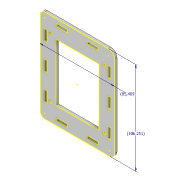
# Autodesk Inventor part: tapa1
Saved by Autodesk Inventor 2019 (Build 230136000, 136)
## iProperties
Created: 2018-09-17
Part Number: tapa1
Material: Genérico
Document SubType Name: Modeling
Designer: lmacia
Density: 1 g/cm^3
Appearance: Valor por defecto
Author: lmacia
Autodesk Inventor part; units mm, degrees
ref_plane "YZ Plane" through (0, 0, 0) normal (1, 0, 0) x (0, 1, 0)
ref_plane "XZ Plane" through (0, 0, 0) normal (0, 1, 0) x (-1, 0, 0)
ref_plane "XY Plane" through (0, 0, 0) normal (0, 0, 1) x (1, 0, 0)
sketch "Boceto1" plane through (0, 0, 0) normal (0, 0, 1) x (-1, 0, 0)
  line L0 (35.0245, 23.8411) -> (34.9228, 23.8411)
  line L1 (34.9228, 23.8411) -> (34.9228, 36.0412)
  line L2 (34.9228, 36.0412) -> (35.0245, 36.0412)
  line L3 (34.9228, 36.0412) -> (37.9729, 36.0412)
  line L4 (38.0745, 36.0412) -> (38.1762, 36.0412)
  line L5 (38.1762, 23.8411) -> (38.0745, 23.8411)
  line L6 (37.9729, 23.8411) -> (34.9228, 23.8411)
  line L7 (34.9937, -6.4559) -> (34.892, -6.4559)
  line L8 (34.892, -6.4559) -> (34.892, 5.7442)
  line L9 (34.892, 5.7442) -> (34.9937, 5.7442)
  line L10 (34.892, 5.7442) -> (38.1762, 5.7442)
  line L11 (38.1762, -6.4559) -> (38.0745, -6.4559)
  line L12 (38.0745, -6.4559) -> (34.9937, -6.4559)
  line L13 (32.3812, 32.3812) -> (32.3327, 32.0128)
  line L14 (32.3327, 32.0128) -> (32.1905, 31.6695)
  line L15 (32.2, 31.6622) -> (31.9738, 31.3674)
  line L16 (31.9643, 31.3747) -> (31.6695, 31.1485)
  line L17 (31.6695, 31.1485) -> (31.3262, 31.0063)
  line L18 (31.3262, 31.0063) -> (30.9578, 30.9578)
  line L19 (30.9578, 30.9578) -> (30.5894, 31.0063)
  line L20 (30.5894, 31.0063) -> (30.2461, 31.1485)
  line L21 (30.2461, 31.1485) -> (29.9513, 31.3747)
  line L22 (29.9418, 31.3674) -> (29.7156, 31.6622)
  line L23 (29.7252, 31.6695) -> (29.583, 32.0128)
  line L24 (29.583, 32.0128) -> (29.5345, 32.3812)
  line L25 (29.5345, 32.3812) -> (29.583, 32.7495)
  line L26 (29.583, 32.7495) -> (29.7252, 33.0928)
  line L27 (29.7252, 33.0928) -> (29.9513, 33.3876)
  line L28 (29.9513, 33.3876) -> (30.2461, 33.6138)
  line L29 (30.2461, 33.6138) -> (30.5894, 33.756)
  line L30 (30.5894, 33.756) -> (30.9578, 33.8045)
  line L31 (30.9594, 33.8164) -> (31.3278, 33.7679)
  line L32 (31.3262, 33.756) -> (31.6695, 33.6138)
  line L33 (31.6695, 33.6138) -> (31.9643, 33.3876)
  line L34 (31.9643, 33.3876) -> (32.1905, 33.0928)
  line L35 (32.1905, 33.0928) -> (32.3327, 32.7495)
  line L36 (32.3327, 32.7495) -> (32.3812, 32.3812)
  line L37 (24.7052, 32.9403) -> (24.7052, -32.9403)
  line L38 (24.7052, -32.9403) -> (-24.7052, -32.9403)
  line L39 (-24.7052, -32.9403) -> (-24.7052, 32.9403)
  line L40 (-24.7052, 32.9403) -> (24.7052, 32.9403)
  line L41 (-35.0245, 36.0412) -> (-34.9228, 36.0412)
  line L42 (-34.9228, 36.0412) -> (-34.9228, 23.8411)
  line L43 (-34.9228, 23.8411) -> (-35.0245, 23.8411)
  line L44 (-35.0245, 23.8411) -> (-38.0745, 23.8411)
  line L45 (-38.0745, 23.8411) -> (-38.1762, 23.8411)
  line L46 (-38.1762, 23.8411) -> (-38.1762, 36.0412)
  line L47 (-38.1762, 36.0412) -> (-38.0745, 36.0412)
  line L48 (-38.0745, 36.0412) -> (-35.0245, 36.0412)
  line L49 (-35.0245, -36.7529) -> (-38.0745, -36.7529)
  line L50 (-38.0745, -36.7529) -> (-38.1762, -36.7529)
  line L51 (-38.1762, -36.7529) -> (-38.1762, -24.5527)
  line L52 (-38.1762, -24.5527) -> (-38.0745, -24.5527)
  line L53 (-38.0745, -24.5527) -> (-35.0245, -24.5527)
  line L54 (-35.0245, -24.5527) -> (-34.9228, -24.5527)
  line L55 (-34.9228, -24.5527) -> (-34.9228, -36.7529)
  line L56 (-34.9228, -36.7529) -> (-35.0245, -36.7529)
  line L57 (-30.5894, 31.0063) -> (-30.9578, 30.9578)
  line L58 (-30.9578, 30.9578) -> (-31.3262, 31.0063)
  line L59 (-31.3262, 31.0063) -> (-31.6695, 31.1485)
  line L60 (-31.6695, 31.1485) -> (-31.9643, 31.3747)
  line L61 (-31.9643, 31.3747) -> (-32.1905, 31.6695)
  line L62 (-32.2016, 31.6649) -> (-32.3438, 32.0082)
  line L63 (-32.3327, 32.0128) -> (-32.3812, 32.3812)
  line L64 (-32.3812, 32.3812) -> (-32.3327, 32.7495)
  line L65 (-32.3327, 32.7495) -> (-32.1905, 33.0928)
  line L66 (-32.1905, 33.0928) -> (-31.9643, 33.3876)
  line L67 (-31.9643, 33.3876) -> (-31.6695, 33.6138)
  line L68 (-31.6695, 33.6138) -> (-31.3262, 33.756)
  line L69 (-31.3262, 33.756) -> (-30.9578, 33.8045)
  line L70 (-30.9562, 33.8164) -> (-30.5878, 33.7679)
  line L71 (-30.5894, 33.756) -> (-30.2461, 33.6138)
  line L72 (-30.2461, 33.6138) -> (-29.9513, 33.3876)
  line L73 (-29.9513, 33.3876) -> (-29.7252, 33.0928)
  line L74 (-29.7252, 33.0928) -> (-29.583, 32.7495)
  line L75 (-29.583, 32.7495) -> (-29.5345, 32.3812)
  line L76 (-29.5345, 32.3812) -> (-29.583, 32.0128)
  line L77 (-29.583, 32.0128) -> (-29.7252, 31.6695)
  line L78 (-29.7252, 31.6695) -> (-29.9513, 31.3747)
  line L79 (-29.9513, 31.3747) -> (-30.2461, 31.1485)
  line L80 (-30.2415, 31.1374) -> (-30.5848, 30.9952)
  line L81 (-38.1762, -6.4559) -> (-38.1762, 5.7442)
  line L82 (-38.1762, 5.7442) -> (-38.0745, 5.7442)
  line L83 (-38.0745, 5.7442) -> (-35.0245, 5.7442)
  line L84 (-35.0245, 5.7442) -> (-34.9228, 5.7442)
  line L85 (-34.9228, 5.7442) -> (-34.9228, -6.4559)
  line L86 (-34.9228, -6.4559) -> (-35.0245, -6.4559)
  line L87 (-35.0245, -6.4559) -> (-38.0745, -6.4559)
  line L88 (-38.0745, -6.4559) -> (-38.1762, -6.4559)
  line L89 (-30.5894, -36.6027) -> (-30.9578, -36.6512)
  line L90 (-30.9578, -36.6512) -> (-31.3262, -36.6027)
  line L91 (-31.3262, -36.6027) -> (-31.6695, -36.4605)
  line L92 (-31.6695, -36.4605) -> (-31.9643, -36.2343)
  line L93 (-31.9643, -36.2343) -> (-32.1905, -35.9395)
  line L94 (-32.2016, -35.9441) -> (-32.3438, -35.6008)
  line L95 (-32.3327, -35.5962) -> (-32.3812, -35.2278)
  line L96 (-32.3812, -35.2278) -> (-32.3327, -34.8595)
  line L97 (-32.3327, -34.8595) -> (-32.1905, -34.5162)
  line L98 (-32.1905, -34.5162) -> (-31.9643, -34.2214)
  line L99 (-31.9643, -34.2214) -> (-31.6695, -33.9952)
  line L100 (-31.6695, -33.9952) -> (-31.3262, -33.853)
  line L101 (-31.3262, -33.853) -> (-30.9578, -33.8045)
  line L102 (-30.9562, -33.7926) -> (-30.5878, -33.8411)
  line L103 (-30.5894, -33.853) -> (-30.2461, -33.9952)
  line L104 (-30.2461, -33.9952) -> (-29.9513, -34.2214)
  line L105 (-29.9513, -34.2214) -> (-29.7252, -34.5162)
  line L106 (-29.7252, -34.5162) -> (-29.583, -34.8595)
  line L107 (-29.583, -34.8595) -> (-29.5345, -35.2278)
  line L108 (-29.5345, -35.2278) -> (-29.583, -35.5962)
  line L109 (-29.583, -35.5962) -> (-29.7252, -35.9395)
  line L110 (-29.7252, -35.9395) -> (-29.9513, -36.2343)
  line L111 (-29.944, -36.2439) -> (-30.2388, -36.4701)
  line L112 (-30.2461, -36.4605) -> (-30.5894, -36.6027)
  line L113 (11.4122, -48.8513) -> (11.4122, -45.8013)
  line L114 (11.4122, -45.8013) -> (11.4122, -45.6996)
  line L115 (11.4122, -45.6996) -> (23.6123, -45.6996)
  line L116 (23.6123, -45.6996) -> (23.6123, -45.8013)
  line L117 (23.6123, -45.8013) -> (23.6123, -48.8513)
  line L118 (23.6123, -48.8513) -> (23.6123, -48.953)
  line L119 (23.6123, -48.953) -> (11.4122, -48.953)
  line L120 (11.4122, -48.953) -> (11.4122, -48.8513)
  line L121 (11.4122, 44.9879) -> (11.4122, 45.0896)
  line L122 (11.4122, 44.9879) -> (11.4122, 48.1396)
  line L123 (11.4122, 48.1396) -> (11.4122, 48.2413)
  line L124 (23.6123, 48.2413) -> (23.6123, 48.1396)
  line L125 (23.6123, 44.9879) -> (11.4122, 44.9879)
  line L126 (-23.6123, 44.9879) -> (-23.6123, 45.0896)
  line L127 (-23.6123, 45.0896) -> (-23.6123, 48.1396)
  line L128 (-23.6123, 48.1396) -> (-23.6123, 48.2413)
  line L129 (-23.6123, 48.2413) -> (-11.4122, 48.2413)
  line L130 (-11.4122, 48.2413) -> (-11.4122, 48.1396)
  line L131 (-11.4122, 48.1396) -> (-11.4122, 45.0896)
  line L132 (-11.4122, 45.0896) -> (-11.4122, 44.9879)
  line L133 (-11.4122, 44.9879) -> (-23.6123, 44.9879)
  line L134 (-11.4122, -45.6996) -> (-11.4122, -45.8013)
  line L135 (-11.4122, -45.8013) -> (-11.4122, -48.8513)
  line L136 (-11.4122, -48.8513) -> (-11.4122, -48.953)
  line L137 (-11.4122, -48.953) -> (-23.6123, -48.953)
  line L138 (-23.6123, -48.953) -> (-23.6123, -48.8513)
  line L139 (-23.6123, -48.8513) -> (-23.6123, -45.8013)
  line L140 (-23.6123, -45.8013) -> (-23.6123, -45.6996)
  line L141 (-23.6123, -45.6996) -> (-11.4122, -45.6996)
  line L142 (32.3327, -34.8595) -> (32.3812, -35.2278)
  line L143 (32.3812, -35.2278) -> (32.3327, -35.5962)
  line L144 (32.3327, -35.5962) -> (32.1905, -35.9395)
  line L145 (32.1905, -35.9395) -> (31.9643, -36.2343)
  line L146 (31.9716, -36.2439) -> (31.6768, -36.4701)
  line L147 (31.6695, -36.4605) -> (31.3262, -36.6027)
  line L148 (31.3262, -36.6027) -> (30.9578, -36.6512)
  line L149 (30.9578, -36.6512) -> (30.5894, -36.6027)
  line L150 (30.5894, -36.6027) -> (30.2461, -36.4605)
  line L151 (30.2461, -36.4605) -> (29.9513, -36.2343)
  line L152 (29.9513, -36.2343) -> (29.7252, -35.9395)
  line L153 (29.7252, -35.9395) -> (29.583, -35.5962)
  line L154 (29.583, -35.5962) -> (29.5345, -35.2278)
  line L155 (29.5345, -35.2278) -> (29.583, -34.8595)
  line L156 (29.583, -34.8595) -> (29.7252, -34.5162)
  line L157 (29.7252, -34.5162) -> (29.9513, -34.2214)
  line L158 (29.944, -34.2118) -> (30.2388, -33.9856)
  line L159 (30.2461, -33.9952) -> (30.5894, -33.853)
  line L160 (30.5894, -33.853) -> (30.9578, -33.8045)
  line L161 (30.9578, -33.8045) -> (31.3262, -33.853)
  line L162 (31.3262, -33.853) -> (31.6695, -33.9952)
  line L163 (31.6768, -33.9856) -> (31.9716, -34.2118)
  line L164 (31.9643, -34.2214) -> (32.1905, -34.5162)
  line L165 (32.1905, -34.5162) -> (32.3327, -34.8595)
  line L166 (34.9228, -36.7529) -> (34.9228, -24.5527)
  line L167 (34.9228, -24.5527) -> (35.0245, -24.5527)
  line L168 (35.0245, -24.5527) -> (38.0745, -24.5527)
  line L169 (38.0745, -24.5527) -> (38.1762, -24.5527)
  line L170 (38.1762, -24.5527) -> (38.1762, -36.7529)
  line L171 (38.1762, -36.7529) -> (38.0745, -36.7529)
  line L172 (38.0745, -36.7529) -> (35.0245, -36.7529)
  line L173 (35.0245, -36.7529) -> (34.9228, -36.7529)
  line L174 (23.6123, -48.953) -> (11.4122, -48.953)
  line L175 (11.4122, -48.953) -> (11.4122, -45.6996)
  line L176 (11.4122, -45.6996) -> (23.6123, -45.6996)
  line L177 (23.6123, -45.6996) -> (23.6123, -48.953)
  line L178 (-11.4122, -48.953) -> (-23.6123, -48.953)
  line L179 (-23.6123, -48.953) -> (-23.6123, -45.6996)
  line L180 (-23.6123, -45.6996) -> (-11.4122, -45.6996)
  line L181 (-11.4122, -45.6996) -> (-11.4122, -48.953)
  line L182 (-34.9228, -36.7529) -> (-38.1762, -36.7529)
  line L183 (-38.1762, -36.7529) -> (-38.1762, -24.5527)
  line L184 (-38.1762, -24.5527) -> (-34.9228, -24.5527)
  line L185 (-34.9228, -24.5527) -> (-34.9228, -36.7529)
  line L186 (-34.9228, -6.4559) -> (-38.1762, -6.4559)
  line L187 (-38.1762, -6.4559) -> (-38.1762, 5.7442)
  line L188 (-38.1762, 5.7442) -> (-34.9228, 5.7442)
  line L189 (-34.9228, 5.7442) -> (-34.9228, -6.4559)
  line L190 (-34.9228, 23.8411) -> (-38.1762, 23.8411)
  line L191 (-38.1762, 23.8411) -> (-38.1762, 36.0412)
  line L192 (-38.1762, 36.0412) -> (-34.9228, 36.0412)
  line L193 (-34.9228, 36.0412) -> (-34.9228, 23.8411)
  line L194 (-23.6123, 44.9879) -> (-11.4122, 44.9879)
  line L195 (-11.4122, 44.9879) -> (-11.4122, 48.2413)
  line L196 (-11.4122, 48.2413) -> (-23.6123, 48.2413)
  line L197 (-23.6123, 48.2413) -> (-23.6123, 44.9879)
  line L198 (11.4122, 44.9879) -> (23.6123, 44.9879)
  line L199 (23.6123, 44.9879) -> (23.6123, 48.2413)
  line L200 (23.6123, 48.2413) -> (11.4122, 48.2413)
  line L201 (11.4122, 48.2413) -> (11.4122, 44.9879)
  line L202 (34.9228, 36.0412) -> (38.1762, 36.0412)
  line L203 (38.1762, 36.0412) -> (38.1762, 23.8411)
  line L204 (38.1762, 23.8411) -> (34.9228, 23.8411)
  line L205 (34.9228, 23.8411) -> (34.9228, 36.0412)
  line L206 (34.892, 5.7442) -> (38.1455, 5.7442)
  line L207 (38.1455, 5.7442) -> (38.1455, -6.4559)
  line L208 (38.1455, -6.4559) -> (34.892, -6.4559)
  line L209 (34.892, -6.4559) -> (34.892, 5.7442)
  line L210 (38.1762, -36.7529) -> (34.9228, -36.7529)
  line L211 (34.9228, -36.7529) -> (34.9228, -24.5527)
  line L212 (34.9228, -24.5527) -> (38.1762, -24.5527)
  line L213 (38.1762, -24.5527) -> (38.1762, -36.7529)
  circle A0 centre (30.9578, 32.3812) radius 1.4232
  circle A1 centre (30.9578, -35.2278) radius 1.4232
  circle A2 centre (-30.9578, -35.2278) radius 1.4232
  circle A3 centre (-30.9578, 32.3812) radius 1.4232
  line L214 (37.2318, -53.5669) -> (-35.5862, -53.5669)
  arc A4 (-42.6187, -46.5344) -> (-35.5862, -53.5669) centre (-35.5862, -46.5344) ccw
  line L215 (-42.6187, -46.5344) -> (-42.6187, 47.1583)
  arc A5 (-37.0932, 52.6838) -> (-42.6187, 47.1583) centre (-37.0932, 47.1583) ccw
  line L216 (-37.0932, 52.6838) -> (37.2318, 52.6838)
  arc A6 (42.7901, 47.1255) -> (37.2318, 52.6838) centre (37.2318, 47.1255) ccw
  line L217 (42.7901, 47.1255) -> (42.7901, -48.0085)
  arc A7 (37.2318, -53.5669) -> (42.7901, -48.0085) centre (37.2318, -48.0085) ccw
  point P0 (0, 0)
  constraints: 436 end point, 20 parallel, 20 tangent, 11 horizontal, 10 perpendicular, 8 centre point, 8 point on circle
extrude "Extrusión1" add sketch "Boceto1" along normal blind 3
sketch "Boceto2" plane through (0, 0, 3) normal (0, 0, 1) x (1, 0, 0)
  line L0 (-24.7052, 32.9403) -> (24.7052, 32.9403) projected
  line L1 (24.7052, 32.9403) -> (24.7052, -32.9403) projected
  line L2 (24.7052, -32.9403) -> (-24.7052, -32.9403) projected
  line L3 (-24.7052, -32.9403) -> (-24.7052, 32.9403) projected
  line L4 (-38.1455, -5.7442) -> (-38.1455, 6.4559) projected
  line L5 (-38.1455, 6.4559) -> (-34.892, 6.4559) projected
  line L6 (-34.892, 6.4559) -> (-34.892, -5.7442) projected
  line L7 (-34.892, -5.7442) -> (-38.1455, -5.7442) projected
  line L8 (-34.9228, 24.5527) -> (-38.1762, 24.5527) projected
  line L9 (-38.1762, 24.5527) -> (-38.1762, 36.7529) projected
  line L10 (-38.1762, 36.7529) -> (-34.9228, 36.7529) projected
  line L11 (-34.9228, 36.7529) -> (-34.9228, 24.5527) projected
  line L12 (23.6123, 48.953) -> (23.6123, 45.6996) projected
  line L13 (23.6123, 45.6996) -> (11.4122, 45.6996) projected
  line L14 (11.4122, 45.6996) -> (11.4122, 48.953) projected
  line L15 (11.4122, 48.953) -> (23.6123, 48.953) projected
  line L16 (11.4122, -44.9879) -> (23.6123, -44.9879) projected
  line L17 (23.6123, -44.9879) -> (23.6123, -48.2413) projected
  line L18 (23.6123, -48.2413) -> (11.4122, -48.2413) projected
  line L19 (11.4122, -48.2413) -> (11.4122, -44.9879) projected
  line L20 (-23.6123, -44.9879) -> (-11.4122, -44.9879) projected
  line L21 (-11.4122, -44.9879) -> (-11.4122, -48.2413) projected
  line L22 (-11.4122, -48.2413) -> (-23.6123, -48.2413) projected
  line L23 (-23.6123, -48.2413) -> (-23.6123, -44.9879) projected
  line L24 (-11.4122, 45.6996) -> (-23.6123, 45.6996) projected
  line L25 (-23.6123, 45.6996) -> (-23.6123, 48.953) projected
  line L26 (-23.6123, 48.953) -> (-11.4122, 48.953) projected
  line L27 (-11.4122, 48.953) -> (-11.4122, 45.6996) projected
  line L28 (38.1762, -5.7442) -> (34.9228, -5.7442) projected
  line L29 (34.9228, -5.7442) -> (34.9228, 6.4559) projected
  line L30 (34.9228, 6.4559) -> (38.1762, 6.4559) projected
  line L31 (38.1762, 6.4559) -> (38.1762, -5.7442) projected
  line L32 (38.1762, 24.5527) -> (34.9228, 24.5527) projected
  line L33 (34.9228, 24.5527) -> (34.9228, 36.7529) projected
  line L34 (34.9228, 36.7529) -> (38.1762, 36.7529) projected
  line L35 (38.1762, 36.7529) -> (38.1762, 24.5527) projected
  line L36 (38.1762, -23.8411) -> (38.1762, -36.0412) projected
  line L37 (38.1762, -36.0412) -> (34.9228, -36.0412) projected
  line L38 (34.9228, -36.0412) -> (34.9228, -23.8411) projected
  line L39 (34.9228, -23.8411) -> (38.1762, -23.8411) projected
  line L40 (-38.1762, -36.0412) -> (-38.1762, -23.8411) projected
  line L41 (-38.1762, -23.8411) -> (-34.9228, -23.8411) projected
  line L42 (-34.9228, -23.8411) -> (-34.9228, -36.0412) projected
  line L43 (-34.9228, -36.0412) -> (-38.1762, -36.0412) projected
  circle A0 centre (30.9578, -32.3812) radius 1.4232 projected
  circle A1 centre (30.9578, 35.2278) radius 1.4232 projected
  circle A2 centre (-30.9578, 35.2278) radius 1.4232 projected
  circle A3 centre (-30.9578, -32.3812) radius 1.4232 projected
  line L44 (35.5862, 53.5669) -> (-37.2318, 53.5669) projected
  arc A4 (-37.2318, 53.5669) -> (-42.7901, 48.0085) centre (-37.2318, 48.0085) ccw projected
  line L45 (-42.7901, 48.0085) -> (-42.7901, -47.1255) projected
  arc A5 (-42.7901, -47.1255) -> (-37.2318, -52.6838) centre (-37.2318, -47.1255) ccw projected
  line L46 (-37.2318, -52.6838) -> (37.0932, -52.6838) projected
  arc A6 (37.0932, -52.6838) -> (42.6187, -47.1583) centre (37.0932, -47.1583) ccw projected
  line L47 (42.6187, -47.1583) -> (42.6187, 46.5344) projected
  arc A7 (42.6187, 46.5344) -> (35.5862, 53.5669) centre (35.5862, 46.5344) ccw projected
  point P0 (0, 0)
  dimension "d12" = 85.4088
  dimension "d13" = 106.2507
  measures "d12" distance between parallel lines of L47 L45
  measures "d13" distance between parallel lines of L46 L44
